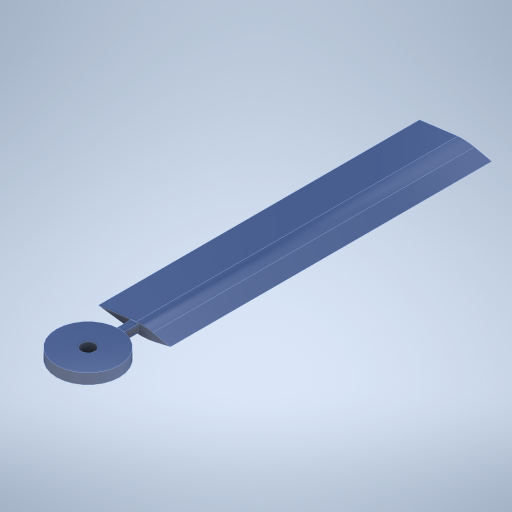
# Autodesk Inventor part: Ruder
Saved by Autodesk Inventor 2023 (Build 270158000, 158)
## iProperties
Created: 2023-05-23
Part Number: Ruder
Material: Generic
Document SubType Name: Modeling
Designer: Sujeet Kumar
Density: 1 g/cm^3
Appearance: Flaked Satin - Blue
Author: Sujeet Kumar
Autodesk Inventor part; units mm, degrees
ref_plane "YZ Plane" through (0, 0, 0) normal (1, 0, 0) x (0, 1, 0)
ref_plane "XZ Plane" through (0, 0, 0) normal (0, 1, 0) x (-1, 0, 0)
ref_plane "XY Plane" through (0, 0, 0) normal (0, 0, 1) x (1, 0, 0)
sketch "Sketch1" plane through (0, 0, 0) normal (0, 0, 1) x (1, 0, 0)
  line L0 (0, 0) -> (55, 0)
  line L1 (0, 0) -> (35, 0)
  line L2 (35, 3.8429) -> (35, 4.5)
  line L3 (29.0376, 3.7334) -> (0, 0)
  line L4 (41.7595, 2.9791) -> (55, 0)
  arc A0 (43.1851, 2.6584) -> (25.4094, 3.2669) centre (32.8243, -40.0614) ccw
  line L5 (-5.4039, 0) -> (70.1536, 0)
  line L6 (0, 0) -> (27.5, 0)
  line L7 (25.4094, 0) -> (29.1094, 0)
  line L8 (29.1094, 0) -> (29.1094, 2.5)
  line L9 (29.1094, 2.5) -> (25.4094, 2.5)
  line L10 (25.4094, 2.5) -> (25.4094, 0)
  dimension "d0" = 55
  dimension "d1" = 35
  dimension "d2" = 4.5
  dimension "d5" = 27.5
  dimension "d6" = 3.7
  dimension "d7" = 2.5
  constraints: 22 end point, 5 point on circle, 5 point on line, 3 horizontal, 2 parallel, 2 perpendicular, 1 centre point
  measures "d0" distance of L0.start L0.end
  measures "d1" distance of L0.start L1.end
  measures "d2" distance of L1.end L2.end
  measures "d5" distance of L0.start L6.end
  measures "d6" distance of L9.end L8.end
  measures "d7" distance of L8.end L7.end
extrude "Extrusion1" add sketch "Sketch1" along normal blind 245 contours L3 A0 L4 L0 L8 L9 L10 | L10 L9 L8 L0
mirror "Mirror1" about plane through (0, 0, 0) normal (0, 1, 0) of "Extrusion1"
sketch "Sketch2" plane through (0, 0, 245) normal (0, 0, 1) x (1, 0, 0)
  line L0 (29.0376, 3.7334) -> (0, 0) projected
  line L1 (0, 0) -> (27.5, 0)
  line L2 (27.5, 0) -> (27.5, 3)
  line L3 (27.5, 3) -> (24.8907, 3)
  line L4 (24.8907, 3) -> (24.8907, -3.2002)
  line L5 (29.0376, -3.7334) -> (0, 0) projected
  line L6 (24.8907, 3) -> (30.3823, 3)
  line L7 (30.3823, 3) -> (30.3823, -3.2002)
  line L8 (30.3823, -3.2002) -> (24.8907, -3.2002)
  line L9 (24.8907, -3.2002) -> (24.8907, 3)
  dimension "d8" = 27.5
  dimension "d9" = 3
  constraints: 16 end point, 4 perpendicular, 2 horizontal, 2 parallel, 1 point on line
  measures "d8" distance of L0.end L1.end
  measures "d9" distance of L1.end L2.end
extrude "Extrusion2" add sketch "Sketch2" along normal blind 10 contours L4 L3 L2 L1 | L1 L2 L6 L7 L8 L4
ref_plane "Work Plane1" through (24.8907, -0.1, 245) normal (0, 1, 0) x (1, 0, 0)
sketch "Sketch3" plane through (24.8907, -0.1, 245) normal (0, 1, 0) x (1, 0, 0)
  line L0 (5.4916, -10) -> (-0.0004, -10)
  line L1 (-0.0004, -10) -> (-0.0004, -35.5)
  line L2 (-0.0004, -35.5) -> (5.4916, -35.5)
  line L3 (5.4916, -35.5) -> (5.4916, -10)
  circle A0 centre (2.7456, -35.5) radius 24
  circle A1 centre (2.7456, -35.5) radius 5.25
  point P0 (-24.8907, 245)
  dimension "d13" = 5.492
  dimension "d14" = 25.5
  dimension "d15" = 48
  dimension "d16" = 10.5
  constraints: 8 end point, 2 centre point, 2 parallel, 1 coincident, 1 horizontal, 1 midpoint, 1 perpendicular
  measures "d13" distance of L2.end L1.end
  measures "d14" distance of L1.end L0.end
  measures "d15" diameter of A0
  measures "d16" diameter of A1
extrude "Extrusion3" add sketch "Sketch3" along normal blind 4 and the other way blind 4 contours A0 L1 A1 L3 | L3 A1 L1 A0
sketch "Sketch4" plane through (0, 0, 255) normal (0, 0, 1) x (1, 0, 0)
  line L0 (24.8907, -3.2002) -> (30.3823, -3.2002) projected
  line L1 (24.8907, 3) -> (24.8907, -3.2002) projected
  line L2 (30.3823, -3.2002) -> (24.8907, -3.2002)
  line L3 (24.8907, -3.2002) -> (24.8907, 3)
  line L4 (24.8907, 3) -> (30.3823, 3)
  line L5 (30.3823, 3) -> (30.3823, -3.2002)
  point P0 (0, 0)
  constraints: 8 end point, 2 parallel, 1 horizontal, 1 perpendicular
extrude "Extrusion4" add sketch "Sketch4" along normal blind 15
body "Solid1"
